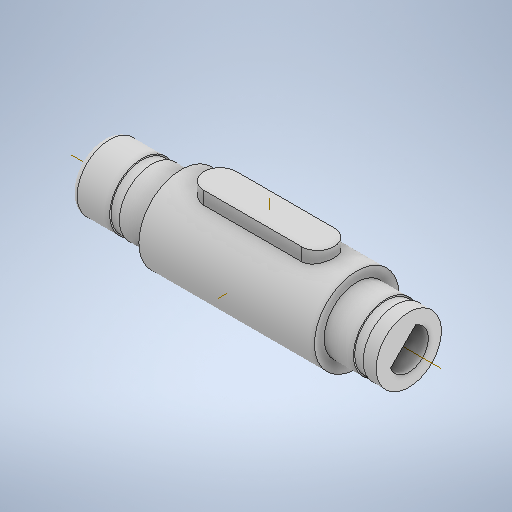
# Autodesk Inventor part: Shaft between link2 and 3
Saved by Autodesk Inventor 2025.2 (Build 292293000, 293)
## iProperties
Created: 2025-03-05
Part Number: Shaft between link2 and 3
Material: Generic
Document SubType Name: Modeling
Designer: abdal
Density: 1 g/cm^3
Appearance: Default
Author: abdal
Autodesk Inventor part; units mm, degrees
ref_plane "YZ Plane" through (0, 0, 0) normal (1, 0, 0) x (0, 1, 0)
ref_plane "XZ Plane" through (0, 0, 0) normal (0, 1, 0) x (-1, 0, 0)
sketch "Sketch1" plane through (0, 0, 0) normal (1, 0, 0) x (0, 1, 0)
  circle A0 centre (0, 0) radius 6.5
  dimension "d0" = 13
  constraints: 1 centre point, 1 coincident
  measures "d0" diameter of A0
extrude "Extrusion1" add sketch "Sketch1" along normal mid plane 27
sketch "Sketch2" plane through (13.5, 0, 0) normal (1, 0, 0) x (0, 0, -1)
  circle A0 centre (0, 0) radius 5
  dimension "d3" = 10
  constraints: 1 centre point, 1 coincident
  measures "d3" diameter of A0
extrude "Extrusion2" add sketch "Sketch2" along normal blind 12
ref_plane "Work Plane1" through (18, 0, 0) normal (1, 0, 0) x (0, 0, -1)
sketch "Sketch3" plane through (18, 0, 0) normal (1, 0, 0) x (0, 0, -1)
  circle A0 centre (0, 0) radius 4.8
  circle A1 centre (0, 0) radius 5 projected
  dimension "d8" = 9.6
  constraints: 1 centre point, 1 coincident
  measures "d8" diameter of A0
extrude "Extrusion3" cut sketch "Sketch3" along normal blind 1.5
mirror "Mirror1" about plane through (0, 0, 0) normal (1, 0, 0) of "Extrusion2", "Extrusion3"
sketch "Sketch4" plane through (0, 0, 0) normal (0, 1, 0) x (-1, 0, 0)
  line L0 (7.5, 0) -> (-7.5, 0) construction
  line L1 (7.5, -2.5) -> (-7.5, -2.5)
  line L2 (-7.5, 2.5) -> (7.5, 2.5)
  arc A0 (7.5, -2.5) -> (7.5, 2.5) centre (7.5, 0) ccw
  arc A1 (-7.5, 2.5) -> (-7.5, -2.5) centre (-7.5, 0) ccw
  point P0 (0, 0)
  point P1 (0, 0)
  point P2 (10, 0)
  point P3 (-10, 0)
  dimension "d11" = 5
  dimension "d12" = 20
  dimension "d13" = 10
  dimension "d14" = 0
  constraints: 8 end point, 6 point on circle, 4 tangent, 2 centre point, 1 horizontal, 1 midpoint, 1 parallel
  measures "d11" distance between parallel lines of L1 L2
  measures "d12" distance of point (10, 0) point (-10, 0)
  measures "d13" distance of point (10, 0) point (0, 0)
  measures "d14" distance of point (0, 0) point (0, 0)
extrude "Extrusion4" add sketch "Sketch4" along normal blind 8
fillet "Fillet2" radius 1 1 edges at (-25.5, 0, 5)
sketch "Sketch6" plane through (25.5, 0, 0) normal (1, 0, 0) x (0, 0, -1)
  circle A0 centre (0, 0) radius 5 projected
extrude "Extrusion6" add sketch "Sketch6" along normal blind 2
sketch "Sketch8" plane through (27.5, 0, 0) normal (1, 0, 0) x (0, 0, -1)
  circle A0 centre (0, 0) radius 3
  line L0 (1.0445, 2.8123) -> (-2.8123, -1.0445)
  line L1 (-2.1213, -2.1213) -> (4.9809, 4.9809)
  line L2 (9.1, 0) -> (-9.1, 0) projected
  point P0 (-0.8839, 0.8839)
  dimension "d30" = 6
  dimension "d31" = 45
  dimension "d32" = 1.25
  constraints: 4 end point, 3 point on circle, 1 centre point, 1 coincident, 1 midpoint, 1 parallel, 1 point on line
  measures "d30" diameter of A0
  measures "d31" angle of L2 L1
  measures "d32" distance of point (0, 0) point (-0.884, 0.884)
extrude "Extrusion8" cut sketch "Sketch8" against normal blind 10.6 contours L0 L2 L1 A0 | L1 L2 A0 | L0 A0 L1 L2 | L2 L1 A0
sketch "Sketch9" plane through (27.5, 0, 0) normal (1, 0, 0) x (0, 0, -1)
  arc A0 (-2.8123, -1.0445) -> (1.0445, 2.8123) centre (0, 0) ccw projected
  line L0 (-2.8123, -1.0445) -> (1.0445, 2.8123) projected
  circle A1 centre (0, 0) radius 5 projected
extrude "Extrusion9" cut sketch "Sketch9" against normal blind 4.6
sketch "Sketch10" plane through (22.9, 0, 0) normal (1, 0, 0) x (0, 0, -1)
  circle A0 centre (0, 0) radius 5 projected
  line L0 (1.0445, 2.8123) -> (-2.8123, -1.0445) projected
  arc A1 (-2.8123, -1.0445) -> (1.0445, 2.8123) centre (0, 0) ccw projected
extrude "Extrusion10" cut sketch "Sketch10" against normal blind 1.4
sketch "Sketch11" plane through (16.9, 0, 0) normal (1, 0, 0) x (0, 0, -1)
  line L0 (-2.8123, -1.0445) -> (1.0445, 2.8123) projected
  arc A0 (-2.8123, -1.0445) -> (1.0445, 2.8123) centre (0, 0) ccw projected
extrude "Extrusion11" cut sketch "Sketch11" against normal up to surface (3.4 mm away)
body "Solid1"
